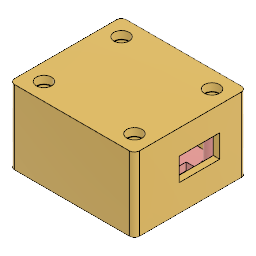
case (Autodesk Fusion 360 design; units mm, degrees)
Autodesk Fusion 360 part; units mm, degrees
note: some values were not read from the file. Set by a fixed rule: which sketch regions a step uses.
sketch "Sketch1" plane through (0, 0, 0) normal (0, 0, 1) x (1, 0, 0)
  line L0 (0, 0) -> (43.18, 0)
  line L1 (43.18, 0) -> (43.18, 38.1)
  line L2 (43.18, 38.1) -> (0, 38.1)
  line L3 (0, 38.1) -> (0, 0)
  line L4 (21.59, 38.1) -> (21.59, 0) construction
  line L5 (0, 19.05) -> (43.18, 19.05) construction
  circle A0 centre (3.81, 34.29) radius 1.45
  circle A1 centre (39.37, 34.29) radius 1.45
  circle A2 centre (39.37, 3.81) radius 1.45
  circle A3 centre (3.81, 3.81) radius 1.45
  circle A4 centre (3.81, 34.29) radius 2.5
  circle A5 centre (39.37, 34.29) radius 2.5
  circle A6 centre (39.37, 3.81) radius 2.5
  circle A7 centre (3.81, 3.81) radius 2.5
  line L6 (43.18, 30.48) -> (33.02, 30.48)
  line L7 (33.02, 30.48) -> (33.02, 14.605)
  line L8 (33.02, 14.605) -> (43.18, 14.605)
  line L9 (0, 30.48) -> (10.16, 30.48)
  line L10 (10.16, 30.48) -> (10.16, 14.605)
  line L11 (10.16, 14.605) -> (0, 14.605)
  dimension "d1" = 43.18
  dimension "d2" = 38.1
  dimension "d3" = 2.9
  dimension "d4" = 35.56
  dimension "d5" = 30.48
  dimension "d6" = 5
  dimension "d11" = 7.62
  dimension "d12" = 10.16
  dimension "d13" = 15.875
  constraint horizontal L0
  constraint vertical L1
  constraint horizontal L2
  constraint vertical L3
  constraint coincident L0.start L3.end
  constraint midpoint L2 L4.start
  constraint midpoint L0 L4.end
  constraint midpoint L3 L5.start
  constraint midpoint L1 L5.end
  constraint symmetric L4 A0 A1
  constraint symmetric L5 A0 A3
  constraint symmetric L5 A1 A2
  constraint concentric A0 A4
  constraint concentric A1 A5
  constraint concentric A2 A6
  constraint concentric A3 A7
  constraint symmetric L4 A4 A5
  constraint symmetric L5 A5 A6
  constraint symmetric L5 A4 A7
  constraint coincident L1 L6.start
  constraint perpendicular L1 L6
  constraint perpendicular L6 L7
  constraint coincident L1 L8.end
  constraint perpendicular L1 L8
  constraint symmetric L4 L6.start L9.start
  constraint symmetric L4 L6.end L9.end
  constraint symmetric L4 L7.end L10.end
  constraint symmetric L4 L8.end L11.end
  measures "d1" distance of L0.start L0.end
  measures "d2" distance of L0.start L2.end
  measures "d3" diameter of A0
  measures "d4" distance of A0.centre A1.centre
  measures "d5" distance of A1.centre A2.centre
  measures "d6" diameter of A4
  measures "d11" distance of L2 L6
  measures "d12" distance of L1 L7
  measures "d13" distance of L6.end L7.end
  measures "d26" distance of L0.end
extrude "Extrude1" add sketch "Sketch1" against normal blind 3 contours L0 L1 L2 L3 L6 L7 L8 L9 L10 L11 | A0 | A1 | A2 | A3 | A4 | A5 | A6 | A7 makes body 1
extrude "Extrude2" add sketch "Sketch1" along normal blind 16.51 contours A4 | A5 | A6 | A7 bodies 1
fillet "Fillet1" radius 1 4 edges at (1.4792, 4.714, 0) (1.4792, 35.194, 0) (37.0392, 35.194, 0) (37.0392, 4.714, 0) on bodies 1
sketch "Sketch2" plane through (0, 0, 16.51) normal (0, 0, 1) x (-1, 0, 0) in component "top"
  circle A0 centre (-39.37, -3.81) radius 1.45
  circle A1 centre (-39.37, -3.81) radius 2.5
  circle A2 centre (-39.37, -34.29) radius 1.45
  circle A3 centre (-39.37, -34.29) radius 2.5
  circle A4 centre (-3.81, -34.29) radius 1.45
  circle A5 centre (-3.81, -34.29) radius 2.5
  circle A6 centre (-3.81, -3.81) radius 1.45
  circle A7 centre (-3.81, -3.81) radius 2.5
  line L0 (-43.18, -30.48) -> (-43.18, -38.1)
  line L1 (-43.18, -38.1) -> (0, -38.1)
  line L2 (0, -38.1) -> (0, -30.48)
  line L3 (0, -30.48) -> (-10.16, -30.48)
  line L4 (-10.16, -30.48) -> (-10.16, -14.605)
  line L5 (-10.16, -14.605) -> (0, -14.605)
  line L6 (0, -14.605) -> (0, 0)
  line L7 (0, 0) -> (-43.18, 0)
  line L8 (-43.18, 0) -> (-43.18, -14.605)
  line L9 (-43.18, -14.605) -> (-33.02, -14.605)
  line L10 (-33.02, -14.605) -> (-33.02, -30.48)
  line L11 (-33.02, -30.48) -> (-43.18, -30.48)
  line L12 (0, -14.605) -> (0, -30.48)
  line L13 (-43.18, -30.48) -> (-43.18, -14.605)
  circle A8 centre (-3.81, -3.81) radius 3
  circle A9 centre (-3.81, -34.29) radius 3
  circle A10 centre (-39.37, -34.29) radius 3
  circle A11 centre (-39.37, -3.81) radius 3
  circle A12 centre (-39.37, -34.29) radius 3.5
  circle A13 centre (-3.81, -3.81) radius 3.5
  circle A14 centre (-3.81, -34.29) radius 3.5
  circle A15 centre (-39.37, -3.81) radius 3.5
  dimension "d19" = 6
  constraint coincident L5.end L6.start
  constraint coincident L2.end L3.start
  constraint coincident L0.start L11.end
  constraint coincident L8.end L9.start
  constraint concentric A6 A8
  constraint equal A8 A9
  constraint equal A8 A11
  constraint equal A10 A11
  measures "d19" diameter of A8
extrude "Extrude1'" add sketch "Sketch2" along normal blind 3 separate body contours A1 | A3 | A5 | A7 makes body 2 at (36.8731, 34.4146, 18.51) makes body 3 at (1.3131, 34.4146, 18.51) makes body 4 at (36.8824, 4.0589, 17.51) makes body 5 at (1.3131, 3.9346, 18.51) in component "top"
extrude "Extrude3" add sketch "Sketch2" along normal blind 2 from surface at 3 contours A1 | A3 | A5 | A7 | A8 | A9 | A10 | A11 bodies 2 3 4 5 in component "top"
extrude "Extrude2'" add sketch "Sketch2" along normal blind 5 from surface at 3 contours L0 L1 L2 L3 L4 L5 L6 L7 L8 L9 L10 L11 | L9 L10 L11 L13 | L3 L4 L5 L12 | A12 | A13 | A14 | A15 bodies 2 3 4 5 in component "top"
move_face "OffsetFaces1" offset -0.3 4 faces at (2.3672, 3.9544, 18.1767) (5.2152, 33.9322, 19.8433) (40.3294, 35.3772, 19.8433) (38.5236, 2.6327, 18.1767) on bodies 2 in component "top"
chamfer "Chamfer1" distance 1 angle 60 4 edges at (5.4416, 3.1772, 21.51) (5.4416, 33.6572, 21.51) (41.0016, 33.6572, 21.51) (41.0016, 3.1772, 21.51) measured on face at (1.2378, 3.661, 21.51) measured on face at (6.3756, 34.054, 21.51) measured on face at (41.9356, 34.054, 21.51) measured on face at (36.8044, 3.574, 21.51) on bodies 2 in component "top"
sketch "Sketch1 (2)" plane through (0, 0, 24.51) normal (0, 0, 1) x (-1, 0, 0) in component "top"
  line L0 (-43.18, -38.1) -> (-43.18, -30.48)
  line L1 (-43.18, -30.48) -> (-33.02, -30.48)
  line L2 (-33.02, -30.48) -> (-33.02, -14.605)
  line L3 (-33.02, -14.605) -> (-43.18, -14.605)
  line L4 (-43.18, -14.605) -> (-43.18, 0)
  line L5 (-43.18, 0) -> (0, 0)
  line L6 (0, 0) -> (0, -14.605)
  line L7 (0, -14.605) -> (-10.16, -14.605)
  line L8 (-10.16, -14.605) -> (-10.16, -30.48)
  line L9 (-10.16, -30.48) -> (0, -30.48)
  line L10 (0, -30.48) -> (0, -38.1)
  line L11 (0, -38.1) -> (-43.18, -38.1)
  line L12 (-43.18, -30.48) -> (-43.18, -14.605)
  line L13 (0, -30.48) -> (0, -14.605)
  line L14 (-43.68, -14.605) -> (-43.68, 0.5)
  line L15 (-43.68, 0.5) -> (0.5, 0.5)
  line L16 (0.5, 0.5) -> (0.5, -14.605)
  line L17 (0.5, -30.48) -> (0.5, -14.605)
  line L18 (0.5, -30.48) -> (0.5, -38.6)
  line L19 (0.5, -38.6) -> (-43.68, -38.6)
  line L20 (-43.68, -38.6) -> (-43.68, -30.48)
  line L21 (-43.68, -30.48) -> (-43.68, -14.605)
  line L22 (-46.18, 3) -> (3, 3)
  line L23 (3, 3) -> (3, -14.605)
  line L24 (3, -30.48) -> (3, -14.605)
  line L25 (3, -30.48) -> (3, -41.1)
  line L26 (3, -41.1) -> (-46.18, -41.1)
  line L27 (-46.18, -41.1) -> (-46.18, -30.48)
  line L28 (-46.18, -30.48) -> (-46.18, -14.605)
  line L29 (-46.18, -14.605) -> (-46.18, 3)
  dimension "d26" = -0.5
  dimension "d27" = -3
  constraint coincident L0.end L1.start
  constraint coincident L3.end L4.start
  constraint coincident L9.end L10.start
  constraint coincident L6.end L7.start
extrude "Extrude5" add sketch "Sketch1 (2)" against normal up to surface (5 mm away) contours L14 L15 L16 L17 L18 L19 L20 L21 bodies 2 in component "top"
extrude "Extrude4" add sketch "Sketch1 (2)" against normal up to surface (29.11 mm away) contours L22 L23 L24 L25 L26 L27 L28 L29 bodies 2 in component "top"
fillet "Fillet1'" radius 2 4 edges at (46.18, -3, 9.955) (-3, -3, 9.955) (-3, 41.1, 9.955) (46.18, 41.1, 9.955) on bodies 2 in component "top"
move_body "Move1" bodies 1 to x (1, 0, 0) y (0, 1, 0) z (0, 0, 1) at (0, 0, -1.6)
sketch "Sketch2 (1)" plane through (-3, 0, 0) normal (-1, 0, 0) x (0, -1, 0) in component "top"
  line L0 (-14.605, -1.6) -> (-30.48, -1.6)
  line L1 (-30.48, -1.6) -> (-30.48, -4.6)
  line L2 (-30.48, -4.6) -> (-14.605, -4.6)
  line L3 (-14.605, -4.6) -> (-14.605, -1.6)
  line L4 (-35.74, 14.91) -> (-32.84, 14.91)
  line L5 (-31.79, 14.91) -> (-36.79, 14.91)
  line L6 (-30.48, 14.91) -> (-14.605, 14.91)
  line L7 (-14.605, 14.91) -> (-14.605, 5.91)
  line L8 (-14.605, 5.91) -> (-30.48, 5.91)
  line L9 (-30.48, 5.91) -> (-30.48, 14.91)
  dimension "d34" = 9
  constraint perpendicular L3 L6
  constraint perpendicular L6 L7
  constraint perpendicular L7 L8
  constraint perpendicular L6 L9
  constraint collinear L1 L9
  constraint collinear L3 L7
  constraint collinear L5 L6
  measures "d34" distance of L6.end L7.end
extrude "Extrude6" cut sketch "Sketch2 (1)" against normal through all contours L6 L7 L8 L9 bodies 2 in component "top"
component "top" placed x (1, 0, 0) y (0, 1, 0) z (0, 0, 1) at (0, 0, 0)
